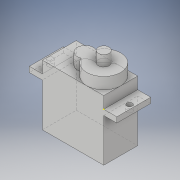
# Autodesk Inventor part: SG92R
Saved by Autodesk Inventor 2017 (Build 210142000, 142)
## iProperties
Created: 2017-06-15
Part Number: SG92R
Material: Generic
Document SubType Name: Modeling
Designer: millerid
Density: 1 g/cm^3
Appearance: Default
Author: millerid
Autodesk Inventor part; units mm, degrees
ref_plane "YZ Plane" through (0, 0, 0) normal (1, 0, 0) x (0, 1, 0)
ref_plane "XZ Plane" through (0, 0, 0) normal (0, 1, 0) x (-1, 0, 0)
ref_plane "XY Plane" through (0, 0, 0) normal (0, 0, 1) x (1, 0, 0)
sketch "Sketch1" plane through (0, 0, 0) normal (0, 1, 0) x (-1, 0, 0)
  line L0 (0, 0) -> (22.8, 0)
  line L1 (22.8, 0) -> (22.8, -12.6)
  line L2 (22.8, -12.6) -> (0, -12.6)
  line L3 (0, -12.6) -> (0, 0)
  dimension "d0" = 22.8
  dimension "d1" = 12.6
  constraints: 8 end point, 2 parallel, 1 horizontal, 1 perpendicular
  measures "d0" distance of L1.end L2.end
  measures "d1" distance of L0.end L1.end
extrude "Extrusion1" add sketch "Sketch1" along normal blind 16
sketch "Sketch2" plane through (0, 16, 0) normal (0, 1, 0) x (1, 0, 0)
  line L0 (0, 0) -> (4.85, 0)
  line L1 (4.85, 0) -> (4.85, 12.6)
  line L2 (0, 12.6) -> (-22.8, 12.6) projected
  line L3 (4.85, 12.6) -> (-22.8, 12.6)
  line L4 (-22.8, 12.6) -> (-27.65, 12.6)
  line L5 (-27.65, 12.6) -> (-27.65, 0)
  line L6 (-27.65, 0) -> (4.85, 0)
  line L7 (-22.8, 0) -> (0, 0) projected
  dimension "d4" = 4.85
  dimension "d5" = 4.85
  constraints: 12 end point, 3 perpendicular, 2 point on line, 1 collinear, 1 horizontal
  measures "d4" distance of L0.start L0.end
  measures "d5" distance of L2.end L4.end
extrude "Extrusion2" add sketch "Sketch2" along normal blind 2
sketch "Sketch3" plane through (0, 18, 0) normal (0, 1, 0) x (1, 0, 0)
  line L0 (-27.65, 0) -> (-22.8, 0) projected
  line L1 (0, 0) -> (0, 12.6) projected
  line L2 (-22.8, 0) -> (0, 0)
  line L3 (0, 0) -> (0, 12.6)
  line L4 (0, 12.6) -> (-22.8, 12.6)
  line L5 (-22.8, 12.6) -> (-22.8, 0)
  constraints: 8 end point, 2 parallel, 1 horizontal, 1 perpendicular
extrude "Extrusion3" add sketch "Sketch3" along normal blind 1
sketch "Sketch4" plane through (0, 18, 0) normal (0, 1, 0) x (1, 0, 0)
  line L0 (-27.65, 12.6) -> (-27.65, 0) projected
  circle A0 centre (-26.09, 6.3) radius 1
  circle A1 centre (3.29, 6.3) radius 1
  line L1 (4.85, 0) -> (4.85, 12.6) projected
  point P0 (0, 0)
  dimension "d11" = 1.56
  dimension "d12" = 2
  dimension "d13" = 2
  dimension "d14" = 1.56
  constraints: 2 centre point
  measures "d11" distance from line of A0.centre L0
  measures "d12" diameter of A0
  measures "d13" diameter of A1
  measures "d14" distance from line of L1 A1.centre
extrude "Extrusion4" cut sketch "Sketch4" against normal through all
sketch "Sketch5" plane through (-27.65, 18, -12.6) normal (0, 1, 0) x (1, 0, 0)
  point P0 (27.65, -12.6)
sketch "Sketch6" plane through (-27.65, 18, -12.6) normal (0, 1, 0) x (1, 0, 0)
  line L0 (4.85, 0) -> (0, 0) projected
  line L1 (4.85, 0) -> (27.65, 0)
  line L2 (27.65, 0) -> (27.65, -12.6)
  line L3 (27.65, -12.6) -> (4.85, -12.6)
  line L4 (4.85, -12.6) -> (4.85, 0)
  constraints: 8 end point, 2 parallel, 1 horizontal, 1 perpendicular
extrude "Extrusion5" add sketch "Sketch6" along normal blind 4.4
sketch "Sketch7" plane through (-27.65, 22.4, -12.6) normal (0, 1, 0) x (1, 0, 0)
  circle A0 centre (21.35, -6.3) radius 6.3
  line L0 (27.65, -12.6) -> (4.85, -12.6) projected
  line L1 (27.65, -12.6) -> (27.65, 0) projected
  circle A1 centre (14.1367, -6.3) radius 3
  dimension "d22" = 6.3
  dimension "d23" = 6
  constraints: 2 centre point, 1 tangent
  measures "d22" distance from line of L1 A0.centre
  measures "d23" diameter of A1
extrude "Extrusion6" add sketch "Sketch7" along normal blind 4.3 contours A0 A1 | A1 A0 picked at (24.082, -5.787) picked at (15.7711, -6.9546)
sketch "Sketch8" plane through (-27.65, 22.4, -12.6) normal (0, 1, 0) x (1, 0, 0)
  circle A0 centre (14.5284, -6.3) radius 3
  point P0 (27.65, -12.6)
  dimension "d26" = 6
  constraints: 1 centre point
  measures "d26" diameter of A0
extrude "Extrusion7" add sketch "Sketch8" along normal blind 4.3
sketch "Sketch9" plane through (-27.65, 26.7, -12.6) normal (0, 1, 0) x (1, 0, 0)
  arc A0 (15.6897, -9.0661) -> (15.6897, -3.5339) centre (21.35, -6.3) ccw projected
  circle A1 centre (21.35, -6.3) radius 2
  point P0 (27.65, -12.6)
  dimension "d29" = 4
  constraints: 1 centre point, 1 coincident
  measures "d29" diameter of A1
extrude "Extrusion8" add sketch "Sketch9" along normal blind 4
body "Solid1"
